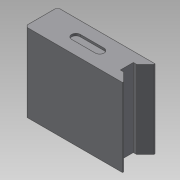
# Autodesk Inventor part: Призма 5
Saved by Autodesk Inventor 2014 SP1 (Build 180222100, 222)
## iProperties
Created: 2014-04-12
Part Number: Призма 5
Material: Типовые
Document SubType Name: Modeling
Designer: Украинцев
Mass: 179.095 g
Surface Area: 232.97 cm^2
Volume: 179.095 cm^3
Density: 1 g/cm^3
Appearance: По умолчанию
Author: Украинцев
Autodesk Inventor part; units mm, degrees
ref_plane "YZ Plane" through (0, 0, 0) normal (1, 0, 0) x (0, 1, 0)
ref_plane "XZ Plane" through (0, 0, 0) normal (0, 1, 0) x (-1, 0, 0)
ref_plane "XY Plane" through (0, 0, 0) normal (0, 0, 1) x (1, 0, 0)
sketch "Эскиз1" plane through (0, 0, 0) normal (0, 0, 1) x (1, 0, 0)
  line L0 (-45, -15) -> (45, -15)
  line L1 (45, 15) -> (-45, 15)
  line L2 (-45, 15) -> (-45, -15)
  line L3 (-45, -15) -> (45, 15) construction
  line L4 (45, -15) -> (-45, 15) construction
  line L5 (45, 14) -> (37, 6)
  line L6 (37, 6) -> (34, 6)
  line L7 (34, 6) -> (34, 0)
  line L8 (34, 0) -> (45, 0) construction
  line L9 (45, -14) -> (37, -6)
  line L10 (37, -6) -> (34, -6)
  line L11 (34, -6) -> (34, 0)
  line L12 (-13, 0) -> (9, 0) construction
  line L13 (-13, -4) -> (9, -4)
  line L14 (9, 4) -> (-13, 4)
  arc A0 (-13, 4) -> (-13, -4) centre (-13, 0) ccw
  arc A1 (9, -4) -> (9, 4) centre (9, 0) ccw
  line L15 (45, -15) -> (45, -14)
  line L16 (45, 14) -> (45, 15)
  circle A2 centre (51.5061, 0) radius 14.5 construction
  point P0 (0, 0)
  point P1 (0, 0)
  point P2 (-2, 0)
  point P3 (0, 0)
  dimension "d0" = 90
  dimension "d1" = 28
  dimension "d2" = 12
  dimension "d3" = 30
  dimension "d4" = 90
  dimension "d5" = 4
  dimension "d6" = 22
  dimension "d7" = 36
  dimension "d9" = 11
  dimension "d17" = 29
  dimension "d18" = 6.5061
  constraints: 36 end point, 6 tangent, 5 midpoint, 5 parallel, 4 point on circle, 3 centre point, 3 perpendicular, 3 symmetric about line, 2 horizontal alignment, 1 horizontal, 1 vertical, 1 vertical alignment
  measures "d0" angle of L9 L5
  measures "d1" distance of L5.start L9.start
  measures "d2" distance between parallel lines of L10 L6
  measures "d3" distance of L1.end L0.start
  measures "d4" distance of L1.start L1.end
  measures "d5" radius of A0
  measures "d6" distance of L12.start L12.end
  measures "d7" distance of L8.end L12.end
  measures "d9" distance between parallel lines of L16 L7
  measures "d17" diameter of A2
  measures "d18" distance from line of A2.centre L16
extrude "Выдавливание1" add sketch "Эскиз1" against normal blind 36 contours L2 L1 L16 L5 L6 L7 L11 L10 L9 L15 L0 | A0 L14 A1 L13
extrude "Выдавливание2" cut sketch "Эскиз1" against normal blind 2 contours A0 L14 A1 L13
mirror "Зеркальное отражение1" about plane through (1.1429, 0, -36) normal (0, 0, -1)
chamfer "Фаска1" distance 2 angle 45 2 edges at (-45, 15, -36) (-45, -15, -36)
